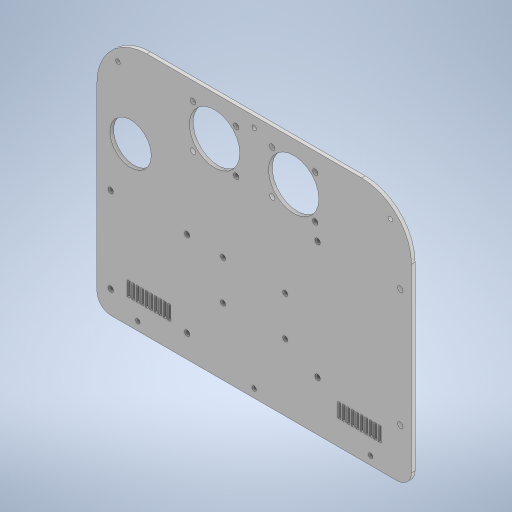
# Autodesk Inventor part: Back_Cover_2
Saved by Autodesk Inventor 2023.5 (Build 275446020, 446B)
## iProperties
Created: 2025-04-17
Part Number: Back_Cover_2
Material: Generic
Document SubType Name: Modeling
Designer: Lucky Sah
Density: 1 g/cm^3
Appearance: Default
Author: Lucky Sah
Autodesk Inventor part; units mm, degrees
ref_plane "YZ Plane" through (0, 0, 0) normal (1, 0, 0) x (0, 1, 0)
ref_plane "XZ Plane" through (0, 0, 0) normal (0, 1, 0) x (-1, 0, 0)
ref_plane "XY Plane" through (0, 0, 0) normal (0, 0, 1) x (1, 0, 0)
sketch "Sketch1" plane through (0, 0, 0) normal (0, 0, 1) x (1, 0, 0)
  line L0 (-119.4404, -59.8278) -> (40.0596, -59.8278)
  line L1 (50.0596, -49.8278) -> (50.0596, 50.6722)
  line L2 (20.0596, 80.6722) -> (-99.4404, 80.6722)
  line L3 (-129.4404, 50.6722) -> (-129.4404, -49.8278)
  arc A0 (50.0596, 50.6722) -> (20.0596, 80.6722) centre (20.0596, 50.6722) ccw
  arc A1 (-99.4404, 80.6722) -> (-129.4404, 50.6722) centre (-99.4404, 50.6722) ccw
  arc A2 (40.0596, -59.8278) -> (50.0596, -49.8278) centre (40.0596, -49.8278) ccw
  arc A3 (-129.4404, -49.8278) -> (-119.4404, -59.8278) centre (-119.4404, -49.8278) ccw
  line L4 (-99.4404, 78.4222) -> (20.0596, 78.4222)
  arc A4 (47.8096, 50.6722) -> (20.0596, 78.4222) centre (20.0596, 50.6722) ccw
  line L5 (47.8096, 50.6722) -> (47.8096, -49.8278)
  arc A5 (40.0596, -57.5778) -> (47.8096, -49.8278) centre (40.0596, -49.8278) ccw
  line L6 (40.0596, -57.5778) -> (-119.4404, -57.5778)
  arc A6 (-127.1904, -49.8278) -> (-119.4404, -57.5778) centre (-119.4404, -49.8278) ccw
  line L7 (-127.1904, -49.8278) -> (-127.1904, 50.6722)
  arc A7 (-99.4404, 78.4222) -> (-127.1904, 50.6722) centre (-99.4404, 50.6722) ccw
  circle A8 centre (36.0596, 66.6722) radius 1.25
  circle A9 centre (-115.4404, 66.6722) radius 1.25
  circle A10 centre (-104.4404, -52.8278) radius 1.25
  circle A11 centre (25.0596, -52.8278) radius 1.25
  circle A12 centre (-39.6904, -52.8278) radius 1.25
  line L8 (-56.9904, 1.6722) -> (-22.3904, 1.6722)
  line L9 (-22.3904, 1.6722) -> (-22.3904, -20.3278)
  line L10 (-22.3904, -20.3278) -> (-56.9904, -20.3278)
  line L11 (-56.9904, -20.3278) -> (-56.9904, 1.6722)
  circle A13 centre (-22.3904, 1.6722) radius 1.375
  circle A14 centre (-56.9904, 1.6722) radius 1.375
  circle A15 centre (-56.9904, -20.3278) radius 1.375
  circle A16 centre (-22.3904, -20.3278) radius 1.375
  line L12 (-119.4904, 2.6722) -> (-76.9904, 2.6722)
  line L13 (-76.9904, 2.6722) -> (-76.9904, -44.8278)
  line L14 (-76.9904, -44.8278) -> (-119.4904, -44.8278)
  line L15 (-119.4904, -44.8278) -> (-119.4904, 2.6722)
  circle A17 centre (-76.9904, 2.6722) radius 1.5
  circle A18 centre (-119.4904, 2.6722) radius 1.5
  circle A19 centre (-119.4904, -44.8278) radius 1.5
  circle A20 centre (-76.9904, -44.8278) radius 1.5
  line L16 (-4.3904, 35.6722) -> (41.6096, 35.6722)
  line L17 (41.6096, 35.6722) -> (41.6096, -29.8278)
  line L18 (41.6096, -29.8278) -> (-4.3904, -29.8278)
  line L19 (-4.3904, -29.8278) -> (-4.3904, 35.6722)
  circle A21 centre (-4.3904, 35.6722) radius 1.5
  circle A22 centre (41.6096, 35.6722) radius 1.5
  circle A23 centre (-4.3904, -29.8278) radius 1.5
  circle A24 centre (41.6096, -29.8278) radius 1.5
  circle A25 centre (-108.4404, 30.6722) radius 11.5
  line L20 (-73.6904, 68.4222) -> (-49.6904, 68.4222)
  line L21 (-49.6904, 68.4222) -> (-49.6904, 44.4222)
  line L22 (-49.6904, 44.4222) -> (-73.6904, 44.4222)
  line L23 (-73.6904, 44.4222) -> (-73.6904, 68.4222)
  line L24 (-29.6904, 68.4222) -> (-5.6904, 68.4222)
  line L25 (-5.6904, 68.4222) -> (-5.6904, 44.4222)
  line L26 (-5.6904, 44.4222) -> (-29.6904, 44.4222)
  line L27 (-29.6904, 44.4222) -> (-29.6904, 68.4222)
  circle A26 centre (-73.6904, 68.4222) radius 1.5
  circle A27 centre (-49.6904, 68.4222) radius 1.5
  circle A28 centre (-73.6904, 44.4222) radius 1.5
  circle A29 centre (-49.6904, 44.4222) radius 1.5
  circle A30 centre (-29.6904, 68.4222) radius 1.5
  circle A31 centre (-5.6904, 68.4222) radius 1.5
  circle A32 centre (-29.6904, 44.4222) radius 1.5
  circle A33 centre (-5.6904, 44.4222) radius 1.5
  line L28 (-39.6904, 78.4222) -> (-39.6904, -57.5778)
  circle A34 centre (-61.6904, 56.4324) radius 14
  circle A35 centre (-17.6904, 56.4324) radius 14
  line L29 (-110.2404, -35.8278) -> (-108.7404, -35.8278)
  line L30 (-108.7404, -35.8278) -> (-108.7404, -43.8278)
  line L31 (-108.7404, -43.8278) -> (-110.2404, -43.8278)
  line L32 (-110.2404, -43.8278) -> (-110.2404, -35.8278)
  line L33 (-107.7404, -35.8278) -> (-106.2404, -35.8278)
  line L34 (-106.2404, -35.8278) -> (-106.2404, -43.8278)
  line L35 (-106.2404, -43.8278) -> (-107.7404, -43.8278)
  line L36 (-107.7404, -43.8278) -> (-107.7404, -35.8278)
  line L37 (-105.2404, -35.8278) -> (-103.7404, -35.8278)
  line L38 (-103.7404, -35.8278) -> (-103.7404, -43.8278)
  line L39 (-103.7404, -43.8278) -> (-105.2404, -43.8278)
  line L40 (-105.2404, -43.8278) -> (-105.2404, -35.8278)
  line L41 (-102.7404, -35.8278) -> (-101.2404, -35.8278)
  line L42 (-101.2404, -35.8278) -> (-101.2404, -43.8278)
  line L43 (-101.2404, -43.8278) -> (-102.7404, -43.8278)
  line L44 (-102.7404, -43.8278) -> (-102.7404, -35.8278)
  line L45 (-100.2404, -35.8278) -> (-98.7404, -35.8278)
  line L46 (-98.7404, -35.8278) -> (-98.7404, -43.8278)
  line L47 (-98.7404, -43.8278) -> (-100.2404, -43.8278)
  line L48 (-100.2404, -43.8278) -> (-100.2404, -35.8278)
  line L49 (-97.7404, -35.8278) -> (-96.2404, -35.8278)
  line L50 (-96.2404, -35.8278) -> (-96.2404, -43.8278)
  line L51 (-96.2404, -43.8278) -> (-97.7404, -43.8278)
  line L52 (-97.7404, -43.8278) -> (-97.7404, -35.8278)
  line L53 (-95.2404, -35.8278) -> (-93.7404, -35.8278)
  line L54 (-93.7404, -35.8278) -> (-93.7404, -43.8278)
  line L55 (-93.7404, -43.8278) -> (-95.2404, -43.8278)
  line L56 (-95.2404, -43.8278) -> (-95.2404, -35.8278)
  line L57 (-92.7404, -35.8278) -> (-91.2404, -35.8278)
  line L58 (-91.2404, -35.8278) -> (-91.2404, -43.8278)
  line L59 (-91.2404, -43.8278) -> (-92.7404, -43.8278)
  line L60 (-92.7404, -43.8278) -> (-92.7404, -35.8278)
  line L61 (-90.2404, -35.8278) -> (-88.7404, -35.8278)
  line L62 (-88.7404, -35.8278) -> (-88.7404, -43.8278)
  line L63 (-88.7404, -43.8278) -> (-90.2404, -43.8278)
  line L64 (-90.2404, -43.8278) -> (-90.2404, -35.8278)
  line L65 (-87.7404, -35.8278) -> (-86.2404, -35.8278)
  line L66 (-86.2404, -35.8278) -> (-86.2404, -43.8278)
  line L67 (-86.2404, -43.8278) -> (-87.7404, -43.8278)
  line L68 (-87.7404, -43.8278) -> (-87.7404, -35.8278)
  line L69 (6.8596, -35.8278) -> (8.3596, -35.8278)
  line L70 (8.3596, -35.8278) -> (8.3596, -43.8278)
  line L71 (8.3596, -43.8278) -> (6.8596, -43.8278)
  line L72 (6.8596, -43.8278) -> (6.8596, -35.8278)
  line L73 (9.3596, -43.8278) -> (9.3596, -35.8278)
  line L74 (10.8596, -43.8278) -> (9.3596, -43.8278)
  line L75 (10.8596, -35.8278) -> (10.8596, -43.8278)
  line L76 (9.3596, -35.8278) -> (10.8596, -35.8278)
  line L77 (11.8596, -43.8278) -> (11.8596, -35.8278)
  line L78 (13.3596, -43.8278) -> (11.8596, -43.8278)
  line L79 (13.3596, -35.8278) -> (13.3596, -43.8278)
  line L80 (11.8596, -35.8278) -> (13.3596, -35.8278)
  line L81 (14.3596, -43.8278) -> (14.3596, -35.8278)
  line L82 (15.8596, -43.8278) -> (14.3596, -43.8278)
  line L83 (15.8596, -35.8278) -> (15.8596, -43.8278)
  line L84 (14.3596, -35.8278) -> (15.8596, -35.8278)
  line L85 (16.8596, -43.8278) -> (16.8596, -35.8278)
  line L86 (18.3596, -43.8278) -> (16.8596, -43.8278)
  line L87 (18.3596, -35.8278) -> (18.3596, -43.8278)
  line L88 (16.8596, -35.8278) -> (18.3596, -35.8278)
  line L89 (19.3596, -43.8278) -> (19.3596, -35.8278)
  line L90 (20.8596, -43.8278) -> (19.3596, -43.8278)
  line L91 (20.8596, -35.8278) -> (20.8596, -43.8278)
  line L92 (19.3596, -35.8278) -> (20.8596, -35.8278)
  line L93 (21.8596, -43.8278) -> (21.8596, -35.8278)
  line L94 (23.3596, -43.8278) -> (21.8596, -43.8278)
  line L95 (23.3596, -35.8278) -> (23.3596, -43.8278)
  line L96 (21.8596, -35.8278) -> (23.3596, -35.8278)
  line L97 (24.3596, -43.8278) -> (24.3596, -35.8278)
  line L98 (25.8596, -43.8278) -> (24.3596, -43.8278)
  line L99 (25.8596, -35.8278) -> (25.8596, -43.8278)
  line L100 (24.3596, -35.8278) -> (25.8596, -35.8278)
  line L101 (26.8596, -43.8278) -> (26.8596, -35.8278)
  line L102 (28.3596, -43.8278) -> (26.8596, -43.8278)
  line L103 (28.3596, -35.8278) -> (28.3596, -43.8278)
  line L104 (26.8596, -35.8278) -> (28.3596, -35.8278)
  line L105 (29.3596, -43.8278) -> (29.3596, -35.8278)
  line L106 (30.8596, -43.8278) -> (29.3596, -43.8278)
  line L107 (30.8596, -35.8278) -> (30.8596, -43.8278)
  line L108 (29.3596, -35.8278) -> (30.8596, -35.8278)
  circle A36 centre (-39.6904, 72.6722) radius 1.25
  point P0 (0, 0)
  point P1 (-129.4404, -59.8278)
  point P2 (50.0596, 0.4222)
  point P3 (-89.4904, -43.8278)
  point P4 (30.8596, -39.8278)
  dimension "d0" = 179.5
  dimension "d1" = 140.5
  dimension "d2" = 30
  dimension "d3" = 10
  dimension "d4" = 2.25
  dimension "d5" = 2.5
  dimension "d6" = 2.5
  dimension "d7" = 2.5
  dimension "d8" = 2.5
  dimension "d9" = 14
  dimension "d10" = 14
  dimension "d11" = 14
  dimension "d12" = 25
  dimension "d13" = 7
  dimension "d14" = 7
  dimension "d15" = 25
  dimension "d16" = 14
  dimension "d17" = 2.5
  dimension "d18" = 7
  dimension "d19" = 89.75
  dimension "d20" = 34.6
  dimension "d21" = 22
  dimension "d22" = 2.75
  dimension "d23" = 2.75
  dimension "d24" = 2.75
  dimension "d25" = 2.75
  dimension "d26" = 72.45
  dimension "d27" = 39.5
  dimension "d28" = 42.5
  dimension "d29" = 47.5
  dimension "d30" = 3
  dimension "d31" = 3
  dimension "d32" = 3
  dimension "d33" = 3
  dimension "d34" = 20
  dimension "d35" = 15
  dimension "d36" = 46
  dimension "d37" = 65.5
  dimension "d38" = 18
  dimension "d39" = 30
  dimension "d40" = 3
  dimension "d41" = 3
  dimension "d42" = 3
  dimension "d43" = 3
  dimension "d44" = 23
  dimension "d45" = 21
  dimension "d46" = 50
  dimension "d49" = 24
  dimension "d50" = 24
  dimension "d51" = 24
  dimension "d52" = 24
  dimension "d53" = 3
  dimension "d54" = 3
  dimension "d55" = 3
  dimension "d56" = 3
  dimension "d57" = 3
  dimension "d58" = 3
  dimension "d59" = 3
  dimension "d60" = 3
  dimension "d61" = 179.5
  dimension "d62" = 10
  dimension "d63" = 20
  dimension "d64" = 20
  dimension "d65" = 28
  constraints: 218 end point, 37 centre point, 20 coincident, 18 parallel, 16 point on circle, 10 horizontal, 9 perpendicular, 8 tangent, 5 midpoint, 4 point on line, 2 collinear, 2 equal radius, 149 other
  measures "d0" distance from line of point (50.06, 0.422) L3
  measures "d1" distance between parallel lines of L0 L2
  measures "d2" radius of A0
  measures "d3" radius of A2
  measures "d4" distance between parallel lines of L2 L4
  measures "d5" diameter of A9
  measures "d6" diameter of A10
  measures "d7" diameter of A11
  measures "d8" diameter of A8
  measures "d9" distance from line of L2 A9.centre
  measures "d10" distance from line of L3 A9.centre
  measures "d11" distance from line of A8.centre L2
  measures "d12" distance from line of L1 A11.centre
  measures "d13" distance from line of L0 A11.centre
  measures "d14" distance from line of L0 A10.centre
  measures "d15" distance from line of L3 A10.centre
  measures "d16" distance from line of L1 A8.centre
  measures "d17" diameter of A12
  measures "d18" distance from line of L0 A12.centre
  measures "d19" distance from line of L1 A12.centre
  measures "d20" distance of L9.end L10.end
  measures "d21" distance of L8.end L9.end
  measures "d22" diameter of A13
  measures "d23" diameter of A14
  measures "d24" diameter of A15
  measures "d25" diameter of A16
  measures "d26" distance between parallel lines of L3 L11
  measures "d27" distance between parallel lines of L0 L10
  measures "d28" distance of L13.end L14.end
  measures "d29" distance of L12.end L13.end
  measures "d30" diameter of A17
  measures "d31" diameter of A18
  measures "d32" diameter of A19
  measures "d33" diameter of A20
  measures "d34" distance between parallel lines of L11 L13
  measures "d35" distance between parallel lines of L0 L14
  measures "d36" distance of L17.end L18.end
  measures "d37" distance of L16.end L17.end
  measures "d38" distance between parallel lines of L9 L19
  measures "d39" distance between parallel lines of L0 L18
  measures "d40" diameter of A21
  measures "d41" diameter of A22
  measures "d42" diameter of A23
  measures "d43" diameter of A24
  measures "d44" diameter of A25
  measures "d45" distance from line of A25.centre L3
  measures "d46" distance from line of A25.centre L2
  measures "d49" distance of L21.end L22.end
  measures "d50" distance of L20.end L21.end
  measures "d51" distance of L25.end L26.end
  measures "d52" distance of L24.end L25.end
  measures "d53" diameter of A26
  measures "d54" diameter of A27
  measures "d55" diameter of A28
  measures "d56" diameter of A29
  measures "d57" diameter of A30
  measures "d58" diameter of A31
  measures "d59" diameter of A32
  measures "d60" diameter of A33
  measures "d61" distance between parallel lines of L1 L3
  measures "d62" distance between parallel lines of L24 L4
  measures "d63" diameter of L27 L28
  measures "d64" diameter of L21 L28
  measures "d65" diameter of A34
extrude "Extrusion1" add sketch "Sketch1" along normal blind 2 contours L4 L28 A36 L8 A14 L11 A15 L10 A12 L6 A6 L7 A7 | L4 A4 L5 A5 L6 L28 A12 L10 A16 L9 A13 L8 A36 | L28 L10 A15 L11 A14 L8 | L8 A13 L9 A16 L10 L28 | L12 A17 L13 A20 L14 A19 L15 A18 | L16 A22 L17 A24 L18 A23 L19 A21 | L20 A34 L23 A26 | L20 A27 L21 A34 | A34 L22 A28 L23 | L21 A29 L22 A34 | L24 A35 L27 A30 | L24 A31 L25 A35 | A35 L26 A32 L27 | L25 A33 L26 A35
body "Solid1"
